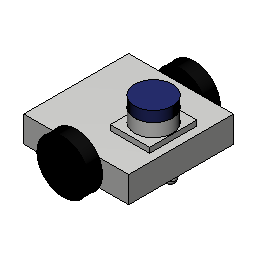
mobile_robot v1 (Autodesk Fusion 360 design; units mm, degrees)
Autodesk Fusion 360 part; units mm, degrees
sketch "Sketch3" plane through (0, 0, 0) normal (0, 0, 1) x (1, 0, 0)
  line L0 (100, 100) -> (-100, 100)
  line L1 (-100, 100) -> (-100, -100)
  line L2 (-100, -100) -> (100, -100)
  line L3 (100, -100) -> (100, 100)
  dimension "d9" = 200
  dimension "d10" = 200
  dimension "d11" = 100
  constraint horizontal L0
  constraint vertical L1
  constraint horizontal L2
  constraint vertical L3
  measures "d9" distance of L0.start L2.end
  measures "d10" distance of L1.end L2.end
  measures "d11" distance of origin L1
extrude "Extrude3" add sketch "Sketch3" along normal blind 50 makes body 1
sketch "Sketch4" plane through (0, -100, 0) normal (0, -1, 0) x (1, 0, 0)
  line L0 (-100, 0) -> (100, 0)
  line L1 (100, 0) -> (100, 50)
  line L2 (100, 50) -> (-100, 50)
  line L3 (-100, 50) -> (-100, 0)
  circle A0 centre (0, 25) radius 50
  dimension "d14" = 100
  dimension "d34" = 25
  measures "d14" diameter of A0
  measures "d34" distance of L0 A0.centre
extrude "Extrude4" add sketch "Sketch4" along normal blind 25 separate body contours L0 L2 A0 | L0 A0 | L2 A0 makes body 2
mirror "Mirror1" about plane through (0, 0, 0) normal (0, 1, 0) of bodies 2 makes body 3
ref_plane "WorkPlane1" through (0, -115.5594, -25) normal (0, 0, -1) x (-1, 0, 0)
move_body "Move1" bodies 3 2 1 to x (1, 0, 0) y (0, 1, 0) z (0, 0, 1) at (0, 0, 25)
sketch "Sketch5" plane through (0, 0, 25) normal (0, 0, -1) x (1, 0, 0)
  line L0 (100, -100) -> (100, 100)
  line L1 (100, 100) -> (-100, 100)
  line L2 (-100, 100) -> (-100, -100)
  line L3 (-100, -100) -> (100, -100)
  circle A0 centre (80, 0) radius 10
  circle A1 centre (-80, 0) radius 10
extrude "Extrude5" add sketch "Sketch5" along normal blind 25 contours A0 | A1 bodies 1
fillet "Fillet1" radius 10 2 edges at (-89.3233, 3.6162, 0) (70.6767, 3.6162, 0) on bodies 1
sketch "Sketch6" plane through (0, 0, 75) normal (0, 0, 1) x (-1, 0, 0)
  line L0 (-100, 100) -> (-100, -100)
  line L1 (-100, -100) -> (100, -100)
  line L2 (100, -100) -> (100, 100)
  line L3 (100, 100) -> (-100, 100)
  line L4 (-10, -45) -> (-85, -45)
  line L5 (-85, -45) -> (-85, 45)
  line L6 (-85, 45) -> (-10, 45)
  line L7 (-10, 45) -> (-10, -45)
  dimension "d24" = 75
  dimension "d25" = 90
  dimension "d26" = 45
  constraint horizontal L4
  constraint vertical L5
  constraint horizontal L6
  constraint vertical L7
  measures "d24" distance of L4.start L4.end
  measures "d25" distance of L4.end L5.end
  measures "d26" distance of origin L4
extrude "Extrude6" add sketch "Sketch6" along normal blind 10 contours L4 L5 L6 L7 bodies 1
sketch "Sketch7" plane through (0, 0, 85) normal (0, 0, 1) x (-1, 0, 0)
  line L0 (-10, 45) -> (-85, 45)
  line L1 (-85, 45) -> (-85, -45)
  line L2 (-85, -45) -> (-10, -45)
  line L3 (-10, -45) -> (-10, 45)
  circle A0 centre (-47.5, 0) radius 36
  dimension "d29" = 72
  measures "d29" diameter of A0
extrude "Extrude7" add sketch "Sketch7" along normal blind 25 contours A0 bodies 1
extrude "Extrude8" add 1 faces at (61.799, 6.0026, 110) along direction (0, 0, 1) blind 20 separate body on bodies 1 makes body 4
copy_body "Body->Comp1" bodies 1 removing the originals makes body 5 in component "base_link"
copy_body "Body->Comp2" bodies 2 removing the originals makes body 6 in component "right_wheel"
copy_body "Body->Comp3" bodies 3 removing the originals makes body 7 in component "left_wheel"
copy_body "Body->Comp4" bodies 4 removing the originals makes body 8 in component "lidar"
component "base_link" placed x (1, 0, 0) y (0, 1, 0) z (0, 0, 1) at (0, 0, 0)
component "right_wheel" placed x (1, 0, 0) y (0, 1, 0) z (0, 0, 1) at (0, 0, 0)
component "left_wheel" placed x (1, 0, 0) y (0, 1, 0) z (0, 0, 1) at (0, 0, 0)
component "lidar" placed x (1, 0, 0) y (0, 1, 0) z (0, 0, 1) at (0, 0, 0)
equation "d26 = ( 90 / 2 ) * 1 mm"
named bodies: "base_link", "right_wheel", "left_wheel", "lidar"
